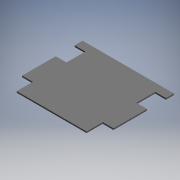
# Autodesk Inventor part: Gen 2.0 rev mecanums base plate
Saved by Autodesk Inventor 2019 (Build 230136000, 136)
## iProperties
Part Number: Gen 2.0 rev mecanums base plate
Material: Generic
Document SubType Name: Modeling
Designer: Delta
Appearance: Default
Author: Delta
Autodesk Inventor part; units mm, degrees
ref_plane "YZ Plane" through (0, 0, 0) normal (1, 0, 0) x (0, 1, 0)
ref_plane "XZ Plane" through (0, 0, 0) normal (0, 1, 0) x (-1, 0, 0)
ref_plane "XY Plane" through (0, 0, 0) normal (0, 0, 1) x (1, 0, 0)
sketch "Sketch1" plane through (0, 0, 0) normal (0, 1, 0) x (-1, 0, 0)
  line L0 (0, 0) -> (431.8, 0)
  line L1 (431.8, 0) -> (431.8, 361.95)
  line L2 (431.8, 361.95) -> (0, 361.95)
  line L3 (0, 361.95) -> (0, 0)
  dimension "d0" = 431.8
  dimension "d1" = 361.95
  constraints: 8 end point, 2 parallel, 1 horizontal, 1 perpendicular
  measures "d0" distance of L1.end L2.end
  measures "d1" distance of L0.end L1.end
extrude "Extrusion1" add sketch "Sketch1" along normal blind 6.35
sketch "Sketch3" plane through (0, 6.35, 0) normal (0, 1, 0) x (1, 0, 0)
  line L0 (-431.8, 0) -> (-431.8, -361.95) projected
  line L1 (-431.8, -361.95) -> (-381, -361.95)
  line L2 (-381, -361.95) -> (-381, -285.75)
  line L3 (-381, -285.75) -> (-431.8, -285.75)
  line L4 (-431.8, -285.75) -> (-431.8, -361.95)
  line L5 (-431.8, -38.1) -> (-381, -38.1)
  line L6 (-381, -38.1) -> (-381, -127)
  line L7 (-381, -127) -> (-431.8, -127)
  line L8 (-431.8, -127) -> (-431.8, -38.1)
  line L9 (0, -361.95) -> (0, 0) projected
  line L10 (0, -38.1) -> (-50.8, -38.1)
  line L11 (-50.8, -38.1) -> (-50.8, -127)
  line L12 (-50.8, -127) -> (0, -127)
  line L13 (0, -127) -> (0, -38.1)
  line L14 (0, -361.95) -> (-50.8, -361.95)
  line L15 (-50.8, -361.95) -> (-50.8, -285.75)
  line L16 (-50.8, -285.75) -> (0, -285.75)
  line L17 (0, -285.75) -> (0, -361.95)
  line L18 (0, 0) -> (-431.8, 0) projected
  dimension "d11" = 76.2
  dimension "d12" = 88.9
  dimension "d13" = 127
  dimension "d14" = 50.8
  dimension "d15" = 50.8
  constraints: 32 end point, 8 parallel, 7 point on line, 4 horizontal, 4 perpendicular
  measures "d11" distance between parallel lines of L1 L3
  measures "d12" distance between parallel lines of L7 L5
  measures "d13" distance between parallel lines of L7 L18
  measures "d14" distance between parallel lines of L2 L4
  measures "d15" distance between parallel lines of L17 L15
extrude "Extrusion3" cut sketch "Sketch3" against normal blind 6.35
body "Solid1"
